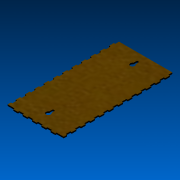
# Autodesk Inventor part: Arriere
Saved by Autodesk Inventor 2013 SP2 (Build 170200200, 200)
## iProperties
Created: 2015-09-16
Part Number: Arriere
Material: Generic
Document SubType Name: Modeling
Designer: jeanfrancois
Density: 1 g/cm^3
Author: jeanfrancois
Autodesk Inventor part; units mm, degrees
ref_plane "YZ Plane" through (0, 0, 0) normal (1, 0, 0) x (0, 1, 0)
ref_plane "XZ Plane" through (0, 0, 0) normal (0, 1, 0) x (-1, 0, 0)
ref_plane "XY Plane" through (0, 0, 0) normal (0, 0, 1) x (1, 0, 0)
sketch "Esquisse1" plane through (0, 0, 0) normal (0, 0, 1) x (1, 0, 0)
  arc A0 (65.5913, 115.695) -> (60.5913, 115.695) centre (63.0913, 115.695) ccw
  line L0 (60.5913, 115.695) -> (60.5913, 110.0251)
  arc A1 (60.5913, 110.0251) -> (65.5913, 110.0251) centre (63.0913, 105.695) ccw
  line L1 (65.5913, 110.0251) -> (65.5913, 115.695)
  arc A2 (65.5913, -64.305) -> (60.5913, -64.305) centre (63.0913, -64.305) ccw
  line L2 (60.5913, -64.305) -> (60.5913, -69.9749)
  arc A3 (60.5913, -69.9749) -> (65.5913, -69.9749) centre (63.0913, -74.305) ccw
  line L3 (65.5913, -69.9749) -> (65.5913, -64.305)
  line L4 (28.0913, -101.305) -> (28.0913, -104.305)
  line L5 (28.0913, -104.305) -> (18.0913, -104.305)
  line L6 (18.0913, -104.305) -> (18.0913, -101.305)
  line L7 (18.0913, -101.305) -> (3.0913, -101.305)
  line L8 (3.0913, -101.305) -> (3.0913, -94.305)
  line L9 (3.0913, -94.305) -> (6.0913, -94.305)
  line L10 (6.0913, -94.305) -> (6.0913, -84.305)
  line L11 (6.0913, -84.305) -> (3.0913, -84.305)
  line L12 (3.0913, -84.305) -> (3.0913, -74.305)
  line L13 (3.0913, -74.305) -> (6.0913, -74.305)
  line L14 (6.0913, -74.305) -> (6.0913, -64.305)
  line L15 (6.0913, -64.305) -> (3.0913, -64.305)
  line L16 (3.0913, -64.305) -> (3.0913, -54.305)
  line L17 (3.0913, -54.305) -> (6.0913, -54.305)
  line L18 (6.0913, -54.305) -> (6.0913, -44.305)
  line L19 (6.0913, -44.305) -> (3.0913, -44.305)
  line L20 (3.0913, -44.305) -> (3.0913, -34.305)
  line L21 (3.0913, -34.305) -> (6.0913, -34.305)
  line L22 (6.0913, -34.305) -> (6.0913, -24.305)
  line L23 (6.0913, -24.305) -> (3.0913, -24.305)
  line L24 (3.0913, -24.305) -> (3.0913, -14.305)
  line L25 (3.0913, -14.305) -> (6.0913, -14.305)
  line L26 (6.0913, -14.305) -> (6.0913, -4.305)
  line L27 (6.0913, -4.305) -> (3.0913, -4.305)
  line L28 (3.0913, -4.305) -> (3.0913, 5.695)
  line L29 (3.0913, 5.695) -> (6.0913, 5.695)
  line L30 (6.0913, 5.695) -> (6.0913, 15.695)
  line L31 (6.0913, 15.695) -> (3.0913, 15.695)
  line L32 (3.0913, 15.695) -> (3.0913, 25.695)
  line L33 (3.0913, 25.695) -> (6.0913, 25.695)
  line L34 (6.0913, 25.695) -> (6.0913, 35.695)
  line L35 (6.0913, 35.695) -> (3.0913, 35.695)
  line L36 (3.0913, 35.695) -> (3.0913, 45.695)
  line L37 (3.0913, 45.695) -> (6.0913, 45.695)
  line L38 (6.0913, 45.695) -> (6.0913, 55.695)
  line L39 (6.0913, 55.695) -> (3.0913, 55.695)
  line L40 (3.0913, 55.695) -> (3.0913, 65.695)
  line L41 (3.0913, 65.695) -> (6.0913, 65.695)
  line L42 (6.0913, 65.695) -> (6.0913, 75.695)
  line L43 (6.0913, 75.695) -> (3.0913, 75.695)
  line L44 (3.0913, 75.695) -> (3.0913, 85.695)
  line L45 (3.0913, 85.695) -> (6.0913, 85.695)
  line L46 (6.0913, 85.695) -> (6.0913, 95.695)
  line L47 (6.0913, 95.695) -> (3.0913, 95.695)
  line L48 (3.0913, 95.695) -> (3.0913, 105.695)
  line L49 (3.0913, 105.695) -> (6.0913, 105.695)
  line L50 (6.0913, 105.695) -> (6.0913, 115.695)
  line L51 (6.0913, 115.695) -> (3.0913, 115.695)
  line L52 (3.0913, 115.695) -> (3.0913, 125.695)
  line L53 (3.0913, 125.695) -> (6.0913, 125.695)
  line L54 (6.0913, 125.695) -> (6.0913, 133.963)
  line L55 (6.0913, 133.963) -> (120.0913, 133.963)
  line L56 (120.0913, 133.963) -> (120.0913, 125.695)
  line L57 (120.0913, 125.695) -> (123.0913, 125.695)
  line L58 (123.0913, 125.695) -> (123.0913, 115.695)
  line L59 (123.0913, 115.695) -> (120.0913, 115.695)
  line L60 (120.0913, 115.695) -> (120.0913, 105.695)
  line L61 (120.0913, 105.695) -> (123.0913, 105.695)
  line L62 (123.0913, 105.695) -> (123.0913, 95.695)
  line L63 (123.0913, 95.695) -> (120.0913, 95.695)
  line L64 (120.0913, 95.695) -> (120.0913, 85.695)
  line L65 (120.0913, 85.695) -> (123.0913, 85.695)
  line L66 (123.0913, 85.695) -> (123.0913, 75.695)
  line L67 (123.0913, 75.695) -> (120.0913, 75.695)
  line L68 (120.0913, 75.695) -> (120.0913, 65.695)
  line L69 (120.0913, 65.695) -> (123.0913, 65.695)
  line L70 (123.0913, 65.695) -> (123.0913, 55.695)
  line L71 (123.0913, 55.695) -> (120.0913, 55.695)
  line L72 (120.0913, 55.695) -> (120.0913, 45.695)
  line L73 (120.0913, 45.695) -> (123.0913, 45.695)
  line L74 (123.0913, 45.695) -> (123.0913, 35.695)
  line L75 (123.0913, 35.695) -> (120.0913, 35.695)
  line L76 (120.0913, 35.695) -> (120.0913, 25.695)
  line L77 (120.0913, 25.695) -> (123.0913, 25.695)
  line L78 (123.0913, 25.695) -> (123.0913, 15.695)
  line L79 (123.0913, 15.695) -> (120.0913, 15.695)
  line L80 (120.0913, 15.695) -> (120.0913, 5.695)
  line L81 (120.0913, 5.695) -> (123.0913, 5.695)
  line L82 (123.0913, 5.695) -> (123.0913, -4.305)
  line L83 (123.0913, -4.305) -> (120.0913, -4.305)
  line L84 (120.0913, -4.305) -> (120.0913, -14.305)
  line L85 (120.0913, -14.305) -> (123.0913, -14.305)
  line L86 (123.0913, -14.305) -> (123.0913, -24.305)
  line L87 (123.0913, -24.305) -> (120.0913, -24.305)
  line L88 (120.0913, -24.305) -> (120.0913, -34.305)
  line L89 (120.0913, -34.305) -> (123.0913, -34.305)
  line L90 (123.0913, -34.305) -> (123.0913, -44.305)
  line L91 (123.0913, -44.305) -> (120.0913, -44.305)
  line L92 (120.0913, -44.305) -> (120.0913, -54.305)
  line L93 (120.0913, -54.305) -> (123.0913, -54.305)
  line L94 (123.0913, -54.305) -> (123.0913, -64.305)
  line L95 (123.0913, -64.305) -> (120.0913, -64.305)
  line L96 (120.0913, -64.305) -> (120.0913, -74.305)
  line L97 (120.0913, -74.305) -> (123.0913, -74.305)
  line L98 (123.0913, -74.305) -> (123.0913, -84.305)
  line L99 (123.0913, -84.305) -> (120.0913, -84.305)
  line L100 (120.0913, -84.305) -> (120.0913, -94.305)
  line L101 (120.0913, -94.305) -> (123.0913, -94.305)
  line L102 (123.0913, -94.305) -> (123.0913, -101.305)
  line L103 (123.0913, -101.305) -> (108.0913, -101.305)
  line L104 (108.0913, -101.305) -> (108.0913, -104.305)
  line L105 (108.0913, -104.305) -> (98.0913, -104.305)
  line L106 (98.0913, -104.305) -> (98.0913, -101.305)
  line L107 (98.0913, -101.305) -> (88.0913, -101.305)
  line L108 (88.0913, -101.305) -> (88.0913, -104.305)
  line L109 (88.0913, -104.305) -> (78.0913, -104.305)
  line L110 (78.0913, -104.305) -> (78.0913, -101.305)
  line L111 (78.0913, -101.305) -> (68.0913, -101.305)
  line L112 (68.0913, -101.305) -> (68.0913, -104.305)
  line L113 (68.0913, -104.305) -> (58.0913, -104.305)
  line L114 (58.0913, -104.305) -> (58.0913, -101.305)
  line L115 (58.0913, -101.305) -> (48.0913, -101.305)
  line L116 (48.0913, -101.305) -> (48.0913, -104.305)
  line L117 (48.0913, -104.305) -> (38.0913, -104.305)
  line L118 (38.0913, -104.305) -> (38.0913, -101.305)
  line L119 (38.0913, -101.305) -> (28.0913, -101.305)
  point P0 (0, 0)
  constraints: 240 end point, 8 point on circle, 4 centre point
extrude "Extrusion1" add sketch "Esquisse1" along normal blind 3
